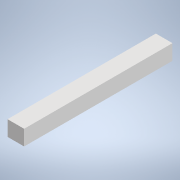
# Autodesk Inventor part: WheelMod
Saved by Autodesk Inventor 2020 (Build 240168000, 168)
## iProperties
Created: 2020-01-19
Part Number: WheelMod
Material: Generic
Document SubType Name: Modeling
Designer: srini
Density: 1 g/cm^3
Appearance: Default
Author: srini
Autodesk Inventor part; units mm, degrees
ref_plane "YZ Plane" through (0, 0, 0) normal (1, 0, 0) x (0, 1, 0)
ref_plane "XZ Plane" through (0, 0, 0) normal (0, 1, 0) x (-1, 0, 0)
sketch "Sketch1" plane through (0, 0, 0) normal (0, 0, 1) x (1, 0, 0)
  line L0 (98.425, -73.787) -> (98.425, -3.937)
  line L1 (184.15, -3.937) -> (184.15, -73.787)
  line L2 (101.6, -78.232) -> (340.5326, -78.232)
  line L3 (98.425, -3.175) -> (184.15, -3.175)
  line L4 (184.15, -3.175) -> (184.15, -78.232)
  line L5 (184.15, -78.232) -> (98.425, -78.232)
  line L6 (98.425, -78.232) -> (98.425, -3.175)
  line L7 (704.85, -3.175) -> (790.575, -3.175)
  line L8 (790.575, -3.175) -> (790.575, -78.232)
  line L9 (790.575, -78.232) -> (704.85, -78.232)
  line L10 (704.85, -78.232) -> (704.85, -3.175)
  line L11 (790.575, -3.937) -> (790.575, -73.787)
  line L12 (704.85, -73.787) -> (704.85, -3.937)
  line L13 (99.187, -3.175) -> (111.125, -3.175)
  point P0 (0, 0)
  constraints: 28 end point, 8 collinear, 4 horizontal, 4 parallel, 4 vertical, 2 perpendicular, 12 other
ref_plane "Work Plane1" through (101.6, -77.47, -820.674) normal (0, 0, -1) x (0, 1, 0)
extrude "Extrusion1" add sketch "Sketch1" against normal up to surface (820.674 mm away)
body "Solid1"
